winged nuts Acryl on small machine_v2 (Autodesk Fusion 360 design; units mm, degrees)
Autodesk Fusion 360 part; units mm, degrees
sketch "nut" plane through (0, 0, 0) normal (0, 0, 1) x (1, 0, 0)
  circle A0 centre (-302, 114) radius 1.05
  circle A1 centre (-154, 222) radius 1.05
  circle A2 centre (-302, 222) radius 1.05
  line L0 (2, 11.8017) -> (42, 11.8017)
  line L1 (42, 11.8017) -> (42, 2)
  line L2 (42, 2) -> (2, 2)
  line L3 (2, 2) -> (2, 11.8017)
  circle A3 centre (22, 6.9008) radius 1.75
  line L4 (2, 6.9008) -> (42, 6.9008)
  spline S0 degree 5 poles (2, 2) (2.4371, 2.1633) (3.3034, 2.4801) (4.5788, 2.9259) (6.2306, 3.4609) (8.2078, 4.0231) (10.0884, 4.4674) (11.8614, 4.7807) (13.5173, 4.9511) (15.0527, 4.9745) (16.4728, 4.8574) (17.5225, 4.6585) (18.2641, 4.4535) (18.7385, 4.2925) (18.9707, 4.2059) knots 0 0 0 0 0 0 0.1 0.2 0.3 0.4 0.5 0.6 0.7 0.8 0.9 1 1 1 1 1 1
  line L5 (22, 11.8017) -> (22, 2)
  spline S1 degree 5 poles (2, 11.8017) (2.4371, 11.6384) (3.3034, 11.3216) (4.5788, 10.8757) (6.2306, 10.3407) (8.2078, 9.7785) (10.0884, 9.3343) (11.8614, 9.021) (13.5173, 8.8506) (15.0527, 8.8272) (16.4728, 8.9443) (17.5225, 9.1432) (18.2641, 9.3482) (18.7385, 9.5092) (18.9707, 9.5958) knots 0 0 0 0 0 0 0.1 0.2 0.3 0.4 0.5 0.6 0.7 0.8 0.9 1 1 1 1 1 1
  line L6 (0.0382, 1.267) -> (3.9618, 2.733)
  line L7 (17.4997, 4.7546) -> (20.4417, 3.6572)
  line L8 (0.0382, 12.5347) -> (3.9618, 11.0687)
  line L9 (17.4997, 9.0471) -> (20.4417, 10.1445)
  spline S2 degree 5 poles (42, 2) (41.5629, 2.1633) (40.6966, 2.4801) (39.4212, 2.9259) (37.7694, 3.4609) (35.7922, 4.0231) (33.9116, 4.4674) (32.1386, 4.7807) (30.4827, 4.9511) (28.9473, 4.9745) (27.5272, 4.8574) (26.4775, 4.6585) (25.7359, 4.4535) (25.2615, 4.2925) (25.0293, 4.2059) knots 0 0 0 0 0 0 0.1 0.2 0.3 0.4 0.5 0.6 0.7 0.8 0.9 1 1 1 1 1 1
  line L10 (43.9618, 1.267) -> (40.0382, 2.733)
  line L11 (26.5003, 4.7546) -> (23.5583, 3.6572)
  spline S3 degree 5 poles (42, 11.8017) (41.5629, 11.6384) (40.6966, 11.3216) (39.4212, 10.8757) (37.7694, 10.3407) (35.7922, 9.7785) (33.9116, 9.3343) (32.1386, 9.021) (30.4827, 8.8506) (28.9473, 8.8272) (27.5272, 8.9443) (26.4775, 9.1432) (25.7359, 9.3482) (25.2615, 9.5092) (25.0293, 9.5958) knots 0 0 0 0 0 0 0.1 0.2 0.3 0.4 0.5 0.6 0.7 0.8 0.9 1 1 1 1 1 1
  line L12 (43.9618, 12.5347) -> (40.0382, 11.0687)
  line L13 (26.5003, 9.0471) -> (23.5583, 10.1445)
  arc A4 (18.9707, 4.2059) -> (25.0293, 4.2059) centre (22, 6.9008) ccw
  arc A5 (25.0293, 9.5958) -> (18.9707, 9.5958) centre (22, 6.9008) ccw
  point P0 (11.2, 0)
  point P1 (12.9999, 4.8785)
  point P2 (12.9999, 8.9232)
  point P3 (31.0001, 4.8785)
  point P4 (31.0001, 8.9232)
  dimension "d488" = 40
  dimension "d495" = 2
  dimension "d497" = 3.5
  dimension "d498" = 8.1092
  constraint horizontal L0
  constraint vertical L1
  constraint horizontal L2
  constraint vertical L3
  constraint midpoint L3 L4.start
  constraint midpoint L1 L4.end
  constraint midpoint A3.centre L4
  constraint concentric A3 A4
  constraint midpoint L0 L5.start
  constraint midpoint L2 L5.end
  constraint midpoint L2.end L6
  constraint midpoint S0.end L7
  constraint symmetric L2.end L4 L0.start
  constraint symmetric L4 P1 P2
  constraint symmetric L4 S0.end S1.end
  constraint symmetric L4 L6.start L8.start
  constraint symmetric L4 L6.end L8.end
  constraint symmetric L4 L7.start L9.start
  constraint symmetric L4 L7.end L9.end
  constraint symmetric L2.end L5 L1.end
  constraint symmetric P1 L5 P3
  constraint symmetric S0.end L5 S2.end
  constraint symmetric L5 L0.start L0.end
  constraint symmetric L5 P2 P4
  constraint symmetric L5 S1.end S3.end
  constraint symmetric L5 L6.start L10.start
  constraint symmetric L5 L6.end L10.end
  constraint symmetric L5 L7.start L11.start
  constraint symmetric L5 L7.end L11.end
  constraint symmetric L5 L8.start L12.start
  constraint symmetric L5 L8.end L12.end
  constraint symmetric L5 L9.start L13.start
  constraint symmetric L5 L9.end L13.end
  constraint concentric A4 A5
  measures "d488" distance of L0.start L0.end
  measures "d495" distance of origin L3
  measures "d497" diameter of A3
  measures "d498" diameter of A4
extrude "Extrude22" add sketch "nut" along normal blind 3.175 contours L3 A3 L4 L5 S1 A5 | L3 A3 L4 S0 L5 A4 | L1 A3 L4 L5 S3 A5 | L1 A3 L4 L5 S2 A4
equation "fingerWidth = 10 mm"
equation "length = 160 mm"
equation "thickness = 3.175 mm"
equation "height = 50 mm"
equation "toolDiameter = 1.401 mm"
equation "boneCornerToCenter = toolDiameter / 2 / sqrt(2) - 0 * kerf" comment "Best: 2.001 -2*kerf, 0.1;;;Best: 2.001 no kerf and 0.1   OLD+6 kerf at 2.001 Diam and .1 mm"
equation "tempLengthPiecesBottom = ceil(( ( floor(( length - 2 * thickness ) / fingerWidth) - 2 ) - ( ( floor(( length - 2 * thickness ) / fingerWidth) - 2 ) % 2 - 1 ) ))"
equation "lengthCutsBottom = ceil(tempLengthPiecesBottom / 2)"
equation "lengthShoulder = ( length - fingerWidth * tempLengthPiecesBottom ) / 2 - kerf"
equation "depth = 120 mm"
equation "tempDepthPiecesBottom = ceil(( ( floor(( depth - 2 * thickness ) / fingerWidth) - 2 ) - ( ( floor(( depth - 2 * thickness ) / fingerWidth) - 2 ) % 2 - 1 ) ))"
equation "depthCutsSideBottom = ceil(tempDepthPiecesBottom / 2)"
equation "depthShoulder = ( depth - fingerWidth * tempDepthPiecesBottom ) / 2 - kerf"
equation "tempHeightPiecesSide = ceil(( ( floor(( height - 2 * thickness ) / fingerWidth) - 2 ) - ( ( floor(( height - 2 * thickness ) / fingerWidth) - 2 ) % 2 - 1 ) ))"
equation "heightCutsSide = ceil(tempHeightPiecesSide / 2)"
equation "heightSholder = ( height - fingerWidth * tempHeightPiecesSide ) / 2 - kerf"
equation "kerf = -0.093 mm"
equation "holeWidth = fingerWidth + 2 * kerf"
equation "lengthShoulderHole = lengthShoulder + 2 * kerf"
equation "depthShouderHole = depthShoulder + 2 * kerf"
equation "heightShoulderHole = heightSholder + 2 * kerf"
equation "assembleScrewDiam = 2.1 mm"
equation "assembleScrewDistance = 6 mm"
equation "assembleAvoidCollisionDistance = 1 mm"
equation "coolingHoleDistance = 8 mm"
equation "boneCornerToCenterPack = -3 * kerf"
equation "boneCornerToCenterSide = boneCornerToCenter - boneCornerToCenterPack"
